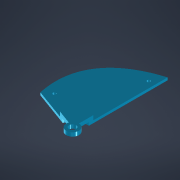
# Autodesk Inventor part: clamshell half-2
Saved by Autodesk Inventor 2021 (Build 250183000, 183)
## iProperties
Created: 2021-02-13
Part Number: clamshell half-2
Material: ABS Plastic
Document SubType Name: Modeling
Designer: vikki
Mass: 5.31327 g
Surface Area: 53.3707 cm^2
Volume: 5.01252 cm^3
Density: 1.06 g/cm^3
Appearance: Sky Blue Dark
Author: vikki
Autodesk Inventor part; units mm, degrees
ref_plane "YZ Plane" through (0, 0, 0) normal (1, 0, 0) x (0, 1, 0)
ref_plane "XZ Plane" through (0, 0, 0) normal (0, 1, 0) x (-1, 0, 0)
ref_plane "XY Plane" through (0, 0, 0) normal (0, 0, 1) x (1, 0, 0)
sketch "Sketch1" plane through (0, 0, 0) normal (0, 1, 0) x (-1, 0, 0)
  circle A0 centre (0, 0) radius 12.5
  line L0 (11.7462, -4.2753) -> (40, -14.5588)
  line L1 (0, 0) -> (41.7481, 0) construction
  line L2 (0, 0) -> (11.7462, -4.2753) construction
  line L3 (0, 0) -> (0, -75)
  line L4 (0, -75) -> (27.0598, -66.8927) construction
  line L5 (27.0598, -66.8927) -> (47.507, -49.1207) construction
  line L6 (47.507, -49.1207) -> (40, -14.5588) construction
  spline S0 degree 3 poles (0, -75) (27.0598, -66.8927) (47.507, -49.1207) (40, -14.5588) knots 1 1 1 1 2 2 2 2
  point P0 (0, -12.5)
  dimension "d0" = 25
  dimension "d1" = 40
  dimension "d3" = 20
  dimension "d4" = 75
  constraints: 8 end point, 1 coincident, 1 collinear, 1 horizontal, 1 vertical, 6 other
  measures "d1" horizontal distance of L0.end point (0, 0)
  measures "d3" angle of L1 L0
  measures "d4" distance of L1.start L3.end
extrude "Extrusion1" add sketch "Sketch1" along normal blind 2
sketch "Sketch2" plane through (0, 0, 0) normal (0, -1, 0) x (1, 0, 0)
  circle A0 centre (0, 0) radius 2.5
  dimension "d7" = 5
  constraints: 1 centre point, 1 coincident
  measures "d7" diameter of A0
extrude "Extrusion2" add sketch "Sketch2" along normal blind 4
sketch "Sketch3" plane through (0, 0, 0) normal (0, -1, 0) x (1, 0, 0)
  arc A0 (11.7462, -4.2753) -> (0, -12.5) centre (0, 0) ccw projected
  arc A1 (0, -12.5) -> (-11.7462, -4.2753) centre (0, 0) ccw projected
extrude "Extrusion3" cut sketch "Sketch3" against normal mid plane 10
sketch "Sketch4" plane through (0, 2, 0) normal (0, 1, 0) x (1, 0, 0)
  circle A0 centre (0, 0) radius 16.5
  arc A1 (0, 12.5) -> (-11.7462, 4.2753) centre (0, 0) ccw projected
  circle A2 centre (0, 0) radius 4.8598
  line L0 (-40, 14.5588) -> (-11.7462, 4.2753) projected
  line L1 (0, 12.5) -> (0, 75) projected
  point P0 (0, 16.5)
  point P1 (-15.5049, 5.6433)
  dimension "d12" = 4
  dimension "d13" = 9.7195
  constraints: 2 centre point, 2 coincident
  measures "d12" radial gap between concentric circles of A0 A1
  measures "d13" diameter of A2
extrude "Extrusion4" add sketch "Sketch4" along normal blind 0.5 contours L1 A1 L0 A0 picked at (-4.9207, 14.2357)
sketch "Sketch5" plane through (0, 2.5, 0) normal (0, 1, 0) x (1, 0, 0)
  circle A0 centre (0, 0) radius 5
  arc A1 (0, 12.5) -> (-11.7462, 4.2753) centre (0, 0) ccw projected
  line L0 (0, 5) -> (0, 12.5)
  line L1 (-11.7462, 4.2753) -> (-4.6985, 1.7101)
  line L2 (-15.5049, 5.6433) -> (-11.7462, 4.2753) projected
  line L3 (0, 12.5) -> (0, 16.5) projected
  arc A2 (0, 16.5) -> (-15.5049, 5.6433) centre (0, 0) ccw projected
  circle A3 centre (0, 0) radius 2.75
  dimension "d16" = 10
  dimension "d17" = 5.5
  constraints: 4 end point, 2 centre point, 2 point on circle, 1 coincident, 1 collinear, 1 vertical
  measures "d16" diameter of A0
  measures "d17" diameter of A3
extrude "Extrusion5" add sketch "Sketch5" along normal blind 3
sketch "Sketch6" plane through (0, 0, 0) normal (0, -1, 0) x (1, 0, 0)
  arc A0 (-11.7462, -4.2753) -> (0, -12.5) centre (0, 0) ccw projected
  line L0 (0, -12.5) -> (0, -75) projected
  line L1 (-40, -14.5588) -> (-11.7462, -4.2753) projected
  circle A1 centre (0, 0) radius 2.75 projected
  circle A2 centre (0, 0) radius 13
  point P0 (-12.216, -4.4463)
  point P1 (0, -13)
  dimension "d20" = 0.5
  constraints: 1 centre point, 1 coincident
  measures "d20" radial gap between concentric circles of A2 A0
extrude "Extrusion6" cut sketch "Sketch6" against normal up to surface (2.5 mm away) contours A0 L0 A2 L1 picked at (-1.0483, -12.7046)
sketch "Sketch7" plane through (0, 0, 0) normal (0, -1, 0) x (1, 0, 0)
  circle A0 centre (-5, -65) radius 1.25
  circle A1 centre (-33.6672, -19.171) radius 1.25
  line L0 (-40, -14.5588) -> (-12.216, -4.4463) projected
  point P0 (0, 0)
  dimension "d23" = 6.5
  dimension "d24" = 19.171
  dimension "d25" = 2.5
  dimension "d26" = 65
  dimension "d27" = 5
  constraints: 2 centre point, 1 equal radius, 1 other
  measures "d23" distance from line of A1.centre L0
  measures "d24" vertical distance of A1.centre point (0, 0)
  measures "d25" diameter of A1
  measures "d26" vertical distance of point (0, 0) A0.centre
  measures "d27" horizontal distance of point (0, 0) A0.centre
extrude "Extrusion7" cut sketch "Sketch7" against normal up to surface (2 mm away)
equation "\"d28\" = d25"
body "Solid1"
